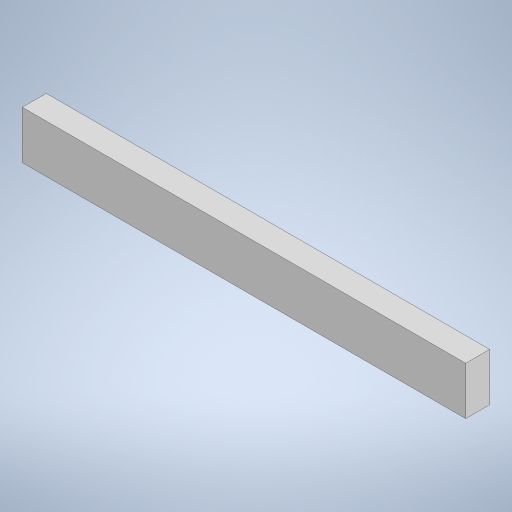
# Autodesk Inventor part: Decal
Saved by Autodesk Inventor 2024 (Build 280153000, 153)
## iProperties
Created: 2023-10-07
Part Number: Decal
Material: Generic
Document SubType Name: Modeling
Designer: chris
Density: 1 g/cm^3
Appearance: Default
Author: chris
Autodesk Inventor part; units mm, degrees
ref_plane "YZ Plane" through (0, 0, 0) normal (1, 0, 0) x (0, 1, 0)
ref_plane "XZ Plane" through (0, 0, 0) normal (0, 1, 0) x (-1, 0, 0)
ref_plane "XY Plane" through (0, 0, 0) normal (0, 0, 1) x (1, 0, 0)
sketch "Sketch1" plane through (0, 0, 0) normal (0, 0, 1) x (1, 0, 0)
  line L0 (-29.56, -3.2) -> (29.56, -3.2)
  line L1 (29.56, -3.2) -> (29.56, 3.2)
  line L2 (29.56, 3.2) -> (-29.56, 3.2)
  line L3 (-29.56, 3.2) -> (-29.56, -3.2)
  line L4 (-29.56, -3.2) -> (29.56, 3.2) construction
  line L5 (29.56, -3.2) -> (-29.56, 3.2) construction
  point P0 (0, 0)
  dimension "d0" = 59.12
  dimension "d1" = 6.4
  constraints: 12 end point, 2 midpoint, 2 parallel, 1 horizontal, 1 perpendicular
  measures "d0" distance of L1.end L2.end
  measures "d1" distance of L0.end L1.end
extrude "Extrusion1" add sketch "Sketch1" along normal blind 3.2
body "Solid1"
